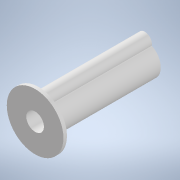
# Autodesk Inventor part: Motorcameralager
Saved by Autodesk Inventor 2021 (Build 250183000, 183)
## iProperties
Created: 2022-06-27
Part Number: Motorcameralager
Material: Generisch
Document SubType Name: Modeling
Designer: adria
Density: 1 g/cm^3
Appearance: Vorgabe
Mass: 1.70726 g
Surface Area: 18.4267 cm^2
Volume: 1.70726 cm^3
Author: adria
Autodesk Inventor part; units mm, degrees
ref_plane "YZ Plane" through (0, 0, 0) normal (1, 0, 0) x (0, 1, 0)
ref_plane "XZ Plane" through (0, 0, 0) normal (0, 1, 0) x (-1, 0, 0)
ref_plane "XY Plane" through (0, 0, 0) normal (0, 0, 1) x (1, 0, 0)
sketch "Skizze1" plane through (0, 0, 0) normal (0, 0, 1) x (1, 0, 0)
  circle A0 centre (0, 0) radius 2.5
  circle A1 centre (0, 0) radius 4.5
  dimension "d0" = 5
  dimension "d1" = 9
  constraints: 2 centre point, 2 coincident
  measures "d0" diameter of A0
  measures "d1" diameter of A1
extrude "Extrusion1" add sketch "Skizze1" along normal blind 30
sketch "Skizze2" plane through (0, 0, 30) normal (0, 0, 1) x (1, 0, 0)
  circle A0 centre (0, 0) radius 4.5 projected
  circle A1 centre (0, 4.5) radius 2
  point P0 (1.95, 4.0556)
  point P1 (-1.95, 4.0556)
  dimension "d4" = 4
  constraints: 1 centre point, 2 other
  measures "d4" diameter of A1
extrude "Extrusion2" add sketch "Skizze2" against normal blind 30 contours A0 A1 picked at (-0.7058, 5.0154)
sketch "Skizze3" plane through (0, 0, 30) normal (0, 0, 1) x (1, 0, 0)
  arc A0 (-1.95, 4.0556) -> (1.95, 4.0556) centre (0, 0) ccw projected
  arc A1 (1.95, 4.0556) -> (-1.95, 4.0556) centre (0, 4.5) ccw projected
  circle A2 centre (0, 0) radius 2.5 projected
  circle A3 centre (0, 0) radius 8
  dimension "d7" = 16
  constraints: 1 centre point, 1 coincident
  measures "d7" diameter of A3
extrude "Extrusion3" add sketch "Skizze3" along normal blind 1 contours A1 A0 | A3
